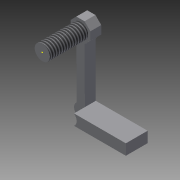
# Autodesk Inventor part: Servo_Arm_Hook
Saved by Autodesk Inventor 2015 SP2 (Build 190223200, 223)
## iProperties
Created: 2016-09-13
Part Number: Servo_Arm_Hook
Material: Generic
Document SubType Name: Modeling
Designer: jm799
Density: 1 g/cm^3
Appearance: Default
Author: jm799
Autodesk Inventor part; units mm, degrees
ref_plane "YZ Plane" through (0, 0, 0) normal (1, 0, 0) x (0, 1, 0)
ref_plane "XZ Plane" through (0, 0, 0) normal (0, 1, 0) x (-1, 0, 0)
ref_plane "XY Plane" through (0, 0, 0) normal (0, 0, 1) x (1, 0, 0)
sketch "Sketch1" plane through (0, 0, 0) normal (0, 1, 0) x (-1, 0, 0)
  circle A0 centre (0, 0) radius 1.4
  dimension "d0" = 2.8
  constraints: 1 centre point, 1 coincident
  measures "d0" diameter of A0
sketch "Sketch2" plane through (0, 0, 0) normal (0, 1, 0) x (-1, 0, 0)
  point P0 (0, 0)
extrude "Extrusion1" add sketch "Sketch1" along normal blind 7
sketch "Sketch3" plane through (0, 7, 0) normal (0, 1, 0) x (1, 0, 0)
  line L0 (1.8253, 0.7457) -> (1.818, -0.7634)
  line L1 (1.818, -0.7634) -> (0.7457, -1.8253)
  line L2 (0.7457, -1.8253) -> (-0.7634, -1.818)
  line L3 (-0.7634, -1.818) -> (-1.8253, -0.7457)
  line L4 (-1.8253, -0.7457) -> (-1.818, 0.7634)
  line L5 (-1.818, 0.7634) -> (-0.7457, 1.8253)
  line L6 (-0.7457, 1.8253) -> (0.7634, 1.818)
  line L7 (0.7634, 1.818) -> (1.8253, 0.7457)
  line L8 (-1.8216, 0.0088) -> (1.8216, -0.0088) construction
  line L9 (-0.0088, -1.8216) -> (0.0088, 1.8216) construction
  point P0 (0, 0)
  point P1 (0, 0)
  point P2 (0, 0)
  point P3 (0, 0)
  constraints: 20 end point, 6 midpoint, 2 coincident, 17 other
extrude "Extrusion2" add sketch "Sketch3" along normal blind 2
sketch "Sketch4" plane through (-0.7457, 7, -1.8253) normal (0.0049, 0, -1) x (-1, 0, -0.0049)
  line L0 (-1.5091, 2) -> (0, 2)
  line L1 (0, 2) -> (0, 0)
  line L2 (0, 0) -> (-1.5091, 0)
  line L3 (-1.5091, 0) -> (-1.5091, 2)
  point P0 (-0.7546, -7)
  constraints: 8 end point, 2 parallel, 1 horizontal, 1 perpendicular
extrude "Extrusion3" add sketch "Sketch4" along normal blind 10
sketch "Sketch5" plane through (0, 9, 0) normal (0, 1, 0) x (1, 0, 0)
  point P0 (0, 0)
sketch "Sketch6" plane through (0, 9, 0) normal (0, 1, 0) x (1, 0, 0)
  point P0 (0, 0)
thread "Thread1" size "M3x0.5" class "6g" standard "ANSI Metric M Profile" full length
sketch "Sketch7" plane through (0, 9, 0) normal (0, 1, 0) x (1, 0, 0)
  circle A0 centre (0.062, 12.7642) radius 1.2414
  point P0 (0, 0)
  constraints: 1 centre point
extrude "Extrusion4" add sketch "Sketch7" against normal blind 2
sketch "Sketch8" plane through (0, 9, 0) normal (0, 1, 0) x (1, 0, 0)
  point P0 (0, 0)
sketch "Sketch9" plane through (0, 9, 0) normal (0, 1, 0) x (1, 0, 0)
  point P0 (0, 0)
sketch "Sketch10" plane through (0, 9, 0) normal (0, 1, 0) x (1, 0, 0)
  line L0 (0.8117, 11.7749) -> (0.8213, 13.7463)
  arc A0 (0.8117, 11.7749) -> (-0.6974, 11.7822) centre (0.062, 12.7642) ccw projected
  line L1 (0.7634, 1.818) -> (0.8117, 11.7749) projected
  line L2 (0.8213, 13.7463) -> (10.3239, 13.7463)
  line L3 (10.3239, 13.7463) -> (10.3239, 11.7749)
  line L4 (10.3239, 11.7749) -> (0.8117, 11.7749)
  line L5 (5.5726, 13.7463) -> (5.5678, 11.7749) construction
  arc A1 (11.8329, 11.7518) -> (10.3238, 11.7518) centre (11.0784, 12.7375) ccw
  arc A2 (10.3238, 11.7518) -> (11.8329, 11.7518) centre (11.0784, 12.7375) ccw
  point P0 (0, 0)
  constraints: 10 end point, 5 point on circle, 3 symmetric about line, 2 centre point, 2 midpoint, 2 perpendicular, 1 collinear, 1 concentric, 1 horizontal, 1 other
extrude "Extrusion5" add sketch "Sketch10" against normal blind 4 contours A0 L2 L3 A1 L4 | A1 L3 L4
sketch "Sketch11" plane through (0, 9, 0) normal (0, 1, 0) x (1, 0, 0)
  point P0 (0, 0)
body "Solid1"
